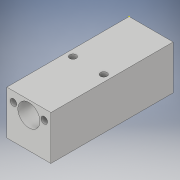
# Autodesk Inventor part: BLOQUE_PRESION
Saved by Autodesk Inventor 2019 (Build 230136000, 136)
## iProperties
Created: 2020-09-15
Part Number: BLOQUE_PRESION
Material: Generic
Document SubType Name: Modeling
Designer: ASUS
Density: 1 g/cm^3
Appearance: Default
Author: ASUS
Autodesk Inventor part; units mm, degrees
ref_plane "YZ Plane" through (0, 0, 0) normal (1, 0, 0) x (0, 1, 0)
ref_plane "XZ Plane" through (0, 0, 0) normal (0, 1, 0) x (-1, 0, 0)
ref_plane "XY Plane" through (0, 0, 0) normal (0, 0, 1) x (1, 0, 0)
sketch "Sketch1" plane through (0, 0, 0) normal (0, 0, 1) x (1, 0, 0)
  line L0 (0, 0) -> (20, 0)
  line L1 (20, 0) -> (20, 20)
  line L2 (20, 20) -> (0, 20)
  line L3 (0, 20) -> (0, 0)
  dimension "d0" = 20
  dimension "d1" = 20
  constraints: 8 end point, 2 parallel, 1 horizontal, 1 perpendicular
  measures "d0" distance of L2.end L1.end
  measures "d1" distance of L1.end L0.end
extrude "Extrusion1" add sketch "Sketch1" along normal blind 55.5
sketch "Sketch2" plane through (0, 0, 0) normal (0, -1, 0) x (1, 0, 0)
  circle A0 centre (17, 28.5) radius 1.5
  circle A1 centre (3, 28.5) radius 1.5
  line L0 (0, 0) -> (20, 0) projected
  dimension "d4" = 14
  dimension "d5" = 3
  dimension "d6" = 28.5
  dimension "d7" = 3
  dimension "d8" = 3
  constraints: 2 centre point, 1 equal radius, 1 horizontal alignment
  measures "d4" distance of A1.centre A0.centre
  measures "d5" diameter of A0
  measures "d6" distance from line of L0 A1.centre
  measures "d7" horizontal distance of L0.end A0.centre
  measures "d8" horizontal distance of L0.start A1.centre
extrude "Extrusion2" cut sketch "Sketch2" against normal through all
sketch "Sketch3" plane through (0, 0, 55.5) normal (0, 0, 1) x (1, 0, 0)
  circle A0 centre (17, 15.5) radius 1.5
  circle A1 centre (3, 15.5) radius 1.5
  line L0 (0, 20) -> (0, 0) projected
  line L1 (20, 0) -> (20, 20) projected
  line L2 (20, 20) -> (0, 20) projected
  dimension "d11" = 3
  dimension "d12" = 3
  dimension "d13" = 14
  dimension "d14" = 3
  dimension "d15" = 3
  dimension "d22" = 4.5
  constraints: 2 centre point, 1 horizontal alignment
  measures "d11" diameter of A0
  measures "d12" diameter of A1
  measures "d13" distance of A1.centre A0.centre
  measures "d14" distance from line of L0 A1.centre
  measures "d15" distance from line of L1 A0.centre
  measures "d22" distance from line of L2 A0.centre
extrude "Extrusion3" cut sketch "Sketch3" against normal blind 10
sketch "Sketch4" plane through (0, 0, 55.5) normal (0, 0, 1) x (1, 0, 0)
  circle A0 centre (10, 14) radius 5
  line L0 (20, 20) -> (0, 20) projected
  point P0 (0, 0)
  point P1 (10, 20)
  dimension "d18" = 6
  dimension "d19" = 10
  constraints: 1 centre point, 1 midpoint, 1 vertical alignment
  measures "d18" distance from line of L0 A0.centre
  measures "d19" diameter of A0
extrude "Extrusion4" cut sketch "Sketch4" against normal through all
sketch "Sketch5" plane through (0, 20, 0) normal (0, 1, 0) x (1, 0, 0)
  point P0 (0, 0)
body "Solid1"
